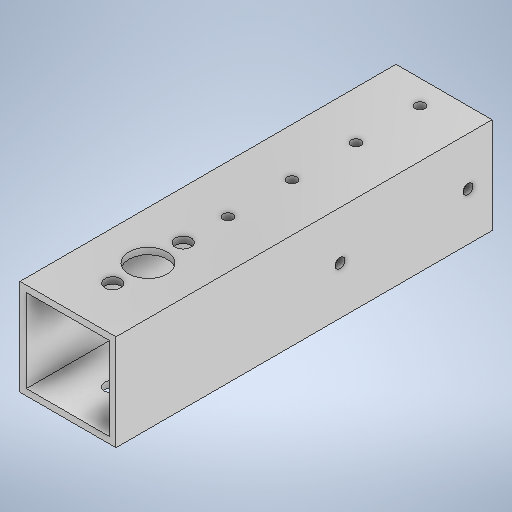
# Autodesk Inventor part: hand2_03
Saved by Autodesk Inventor 2025.1 (Build 291241000, 241)
## iProperties
Created: 2025-02-02
Part Number: hand2_03
Material: アルミニウム 6061-AHC
Document SubType Name: Modeling
Designer: ryogo
Density: 2.7 g/cm^3
Appearance: アルミニウム - ダーク
Author: ryogo
Autodesk Inventor part; units mm, degrees
ref_plane "YZ Plane" through (0, 0, 0) normal (1, 0, 0) x (0, 1, 0)
ref_plane "XZ Plane" through (0, 0, 0) normal (0, 1, 0) x (-1, 0, 0)
ref_plane "XY Plane" through (0, 0, 0) normal (0, 0, 1) x (1, 0, 0)
sketch "スケッチ1" plane through (0, 0, 0) normal (0, 1, 0) x (-1, 0, 0)
  circle A0 centre (0, 0) radius 122.5
  line L0 (0, 0) -> (21.2719, 120.6389)
  line L1 (21.2719, 120.6389) -> (-21.2719, -120.6389)
  line L2 (21.2719, 120.6389) -> (-41.166, -233.4643)
  arc A1 (21.2719, 120.6389) -> (0, 122.5) centre (0, 0) ccw
  arc A2 (-21.2719, -120.6389) -> (0, -122.5) centre (0, 0) ccw
  arc A3 (-41.8975, -115.1123) -> (-21.2719, -120.6389) centre (0, 0) ccw
  circle A4 centre (0, 0) radius 125
  circle A5 centre (0, 0) radius 145
  arc A6 (-42.7525, -117.4616) -> (-105.9051, -66.4011) centre (0, 0) ccw
  line L3 (0, 0) -> (-42.7525, -117.4616) construction
  line L4 (21.706, 123.101) -> (21.706, 123.101)
  line L5 (0, -145) -> (0, -265.735)
  line L6 (0, 0) -> (-41.8975, -115.1123)
  line L7 (-49.5929, -136.2554) -> (-41.8975, -115.1123)
  line L8 (-42.7525, -117.4616) -> (-231.4975, -48.764)
  line L9 (42.7525, 117.4616) -> (0, 0)
  line L10 (0, -145) -> (0, 145)
  line L11 (0, 0) -> (0, 250)
  circle A7 centre (0, 250) radius 20
  line L12 (113.4405, 52.5) -> (18.1505, 258.4)
  line L13 (0, 0) -> (185.4327, 0)
  line L14 (0, 0) -> (-259.4726, 94.4403)
  line L15 (42.7525, 117.4616) -> (-253.7236, 225.3701)
  line L16 (0, 125) -> (22.0409, 125)
  line L17 (21.2719, 120.6389) -> (25.179, 142.7971)
  line L18 (42.7525, 117.4616) -> (60.6365, 166.5974)
  line L19 (15, 170) -> (59.0618, 170)
  line L20 (15.9946, 175) -> (56.7478, 175)
  line L21 (0, 125) -> (-15, 125)
  line L22 (-15, 125) -> (-15, 275)
  line L23 (-15, 275) -> (0, 275)
  line L24 (0, 275) -> (0, 125)
  line L25 (0, 125) -> (15, 125)
  line L26 (15, 125) -> (15, 275)
  line L27 (15, 275) -> (0, 275)
  line L28 (0, 275) -> (0, 125)
  line L29 (15, 200) -> (15, 275)
  line L30 (15, 275) -> (-15, 275)
  line L31 (-15, 275) -> (-15, 150)
  line L32 (15, 170) -> (37.5, 170)
  line L33 (37.5, 170) -> (17.5, 170)
  line L34 (0, 0) -> (0, 250)
  line L35 (0, -125) -> (42.7525, 117.4616)
  line L36 (-42.7525, -117.4616) -> (0, 125)
  line L37 (0, -125) -> (-3.519, -144.9573)
  line L38 (42.7525, 117.4616) -> (49.5929, 136.2554)
  line L39 (0, 125) -> (3.519, 144.9573)
  line L40 (-42.7525, -117.4616) -> (-46.2715, -137.4189)
  line L41 (42.7525, 117.4616) -> (46.2715, 137.4189)
  line L42 (-3.519, -144.9573) -> (46.2715, 137.4189)
  line L43 (46.2715, 137.4189) -> (37.2054, 139.0175)
  line L44 (-12.5852, -143.3587) -> (-3.519, -144.9573)
  line L45 (-46.2715, -137.4189) -> (3.519, 144.9573)
  line L46 (3.519, 144.9573) -> (12.5852, 143.3587)
  line L47 (-37.2054, -139.0175) -> (-46.2715, -137.4189)
  line L48 (-27.6373, -142.3418) -> (-22.7132, -143.21)
  line L49 (-27.6373, -142.3418) -> (-22.7132, -143.21)
  line L50 (-22.7132, -143.21) -> (27.641, 142.363)
  line L51 (27.641, 142.363) -> (22.717, 143.2312)
  line L52 (22.717, 143.2312) -> (-27.6373, -142.3418)
  line L53 (12.5852, 143.3587) -> (-37.2054, -139.0175)
  line L54 (-12.5852, -143.3587) -> (37.2054, 139.0175)
  line L55 (-42.1294, -138.1492) -> (7.6611, 144.2269)
  line L56 (-7.6611, -144.2269) -> (42.1294, 138.1492)
  line L57 (12.5852, 143.3587) -> (7.6611, 144.2269)
  line L58 (7.6611, 144.2269) -> (23.8851, 236.2374)
  line L59 (23.8851, 236.2374) -> (28.8091, 235.3692)
  line L60 (28.8091, 235.3692) -> (12.5852, 143.3587)
  line L61 (22.717, 143.2312) -> (25.179, 142.7971)
  line L62 (25.179, 142.7971) -> (42.462, 240.8141)
  line L63 (42.462, 240.8141) -> (40, 241.2482)
  line L64 (40, 241.2482) -> (22.717, 143.2312)
  line L65 (42.1294, 138.1492) -> (37.2054, 139.0175)
  line L66 (37.2054, 139.0175) -> (45.9435, 188.5741)
  line L67 (45.9435, 188.5741) -> (50.8676, 187.7058)
  line L68 (50.8676, 187.7058) -> (42.1294, 138.1492)
  line L69 (25.179, 142.7971) -> (27.641, 142.363)
  line L70 (27.641, 142.363) -> (39.8383, 211.5375)
  line L71 (39.8383, 211.5375) -> (37.3763, 211.9716)
  line L72 (37.3763, 211.9716) -> (25.179, 142.7971)
  line L73 (15.9946, 175) -> (15, 175)
  line L74 (15, 175) -> (0, 175)
  line L75 (0, 175) -> (0, 170)
  line L76 (0, 170) -> (15, 170)
  line L77 (15, 170) -> (15, 175)
  line L78 (20, 175) -> (40, 175)
  line L79 (40, 175) -> (40, 245)
  line L80 (40, 245) -> (20, 245)
  line L81 (20, 245) -> (20, 175)
  line L82 (30, 175) -> (30, 118.7697)
  line L83 (0, 175) -> (45.1779, 175)
  line L84 (45.1779, 175) -> (45.1779, 200)
  line L85 (45.1779, 200) -> (0, 200)
  line L86 (0, 200) -> (0, 175)
  line L87 (0, 200) -> (50, 200)
  line L88 (50, 200) -> (50, 170)
  line L89 (50, 170) -> (0, 170)
  line L90 (0, 170) -> (0, 200)
  line L91 (50, 170) -> (0, 170)
  line L92 (0, 170) -> (0, 165)
  line L93 (0, 200) -> (-15, 200)
  line L94 (-15, 200) -> (-15, 180)
  line L95 (-15, 180) -> (0, 180)
  line L96 (0, 180) -> (0, 200)
  line L97 (0, 180) -> (-15, 180)
  line L98 (-15, 180) -> (-15, 175)
  line L99 (-15, 175) -> (0, 175)
  line L100 (0, 175) -> (0, 180)
  line L101 (0, 145) -> (-15, 145)
  line L102 (-15, 145) -> (-20.5, 145)
  line L103 (-20.5, 145) -> (-20.5, 200)
  line L104 (-20.5, 200) -> (-15, 200)
  line L105 (-15, 200) -> (-15, 145)
  line L106 (-20.5, 150) -> (-25, 150)
  line L107 (-25, 150) -> (-25, 180)
  line L108 (-25, 180) -> (-20.5, 180)
  line L109 (-20.5, 180) -> (-20.5, 150)
  line L110 (50, 175) -> (-15, 175)
  line L111 (-15, 175) -> (-15, 170)
  line L112 (50, 170) -> (50, 175)
  line L113 (-20.5, 165) -> (-25, 165)
  line L114 (-25, 165) -> (-25, 195)
  line L115 (-25, 195) -> (-20.5, 195)
  line L116 (-20.5, 195) -> (-20.5, 165)
  line L117 (15, 250) -> (-15, 250)
  line L118 (-15, 145) -> (15, 145)
  line L119 (26.3471, 235.8033) -> (-39.6674, -138.5834)
  line L120 (48.4056, 188.14) -> (-10.1232, -143.7928)
  line L121 (49.3441, 179.0659) -> (14.8758, 185.1436)
  line L122 (-15, 138.4818) -> (-15, 121.5782)
  line L123 (-7.6611, -144.2269) -> (-42.1294, -138.1492)
  line L124 (-39.6243, -123.9424) -> (-5.1561, -130.02)
  line L125 (-42.2291, -138.7145) -> (-7.7608, -144.7922)
  line L126 (-41.3608, -133.7904) -> (-6.8926, -139.8681)
  line L127 (-6.0243, -134.9441) -> (-40.4926, -128.8664)
  line L128 (18.3488, 204.8397) -> (52.8171, 198.762)
  line L129 (50.2124, 183.9899) -> (45.0029, 154.4457)
  line L130 (10.5346, 160.5234) -> (15.7441, 190.0676)
  line L131 (19.217, 209.7638) -> (53.6853, 203.6861)
  line L132 (15, 250) -> (53.6853, 203.6861)
  line L133 (53.6853, 203.6861) -> (53.6853, 170)
  line L134 (53.6853, 170) -> (-15, 170)
  line L135 (-15, 172.5) -> (53.6853, 172.5)
  line L136 (15, 170) -> (15, 150)
  line L137 (15, 150) -> (-15, 150)
  line L138 (-15, 170) -> (15, 170)
  line L139 (15, 150) -> (-15, 150)
  line L140 (-15, 150) -> (-15, 275)
  line L141 (-15, 275) -> (15, 275)
  line L142 (15, 275) -> (15, 150)
  circle A8 centre (0, 250) radius 6
  circle A9 centre (0, 250) radius 11
  line L143 (47.7456, 170) -> (15, 150)
  point P0 (-25.1752, -142.7759)
  point P1 (42.3116, 114.9608)
  point P2 (0, 133.0222)
  point P3 (-38.8988, -134.2246)
  point P4 (-38.0306, -129.3005)
  point P5 (-23.2585, -131.9052)
  point P6 (-24.1267, -136.8293)
  point P7 (-9.3546, -139.434)
  point P8 (-8.4863, -134.51)
  point P9 (17.3379, 184.7094)
  point P10 (32.11, 182.1047)
  point P11 (46.8821, 179.5)
  point P12 (50.3551, 199.1962)
  point P13 (35.5829, 201.8009)
  point P14 (20.8108, 204.4056)
  point P15 (0, 240)
  point P16 (0, 190)
  point P17 (0, 239)
  point P18 (0, 261)
  point P19 (37.5, 172.5)
  point P20 (22.5, 172.5)
  point P21 (0, 275)
  point P22 (15, 185.1217)
  point P23 (15, 185.8477)
  point P24 (-11, 250)
  point P25 (11, 250)
  dimension "d0" = 245
  dimension "d7" = 290
  dimension "d19" = 40
  dimension "d1" = 0
  dimension "d4" = 42.5438
  dimension "d5" = 21.3532
  dimension "d6" = 250
  dimension "d10" = 0
  dimension "d12" = 0
  dimension "d13" = 10
  dimension "d15" = 0
  dimension "d16" = 9.8877
  dimension "d18" = 10
  dimension "d21" = 145
  dimension "d23" = 125
  dimension "d26" = 7.5384
  dimension "d30" = 180
  dimension "d34" = 180
  dimension "d35" = 45
  dimension "d37" = 5
  dimension "d38" = 15
  dimension "d39" = 150
  dimension "d40" = 15
  dimension "d41" = 150
  dimension "d47" = 250
  dimension "d52" = 5
  dimension "d53" = 0
  dimension "d54" = 10
  dimension "d55" = 10
  dimension "d56" = 5
  dimension "d57" = 5
  dimension "d60" = 5
  dimension "d61" = 20
  dimension "d62" = 70
  dimension "d63" = 5
  dimension "d65" = 25
  dimension "d66" = 50
  dimension "d68" = 20
  dimension "d69" = 5
  dimension "d74" = 20
  dimension "d75" = 5.5
  dimension "d76" = 55
  dimension "d77" = 4.5
  dimension "d78" = 30
  dimension "d79" = 5
  dimension "d82" = 15
  dimension "d83" = 50
  dimension "d87" = 16.9036
  dimension "d88" = 10.0392
  dimension "d89" = 10.5222
  dimension "d92" = 15
  dimension "d93" = 5
  dimension "d94" = 5
  dimension "d96" = 4.5
  dimension "d97" = 5
  dimension "d98" = 30
  dimension "d99" = 10
  dimension "d101" = 20
  dimension "d102" = 10
  dimension "d103" = 20
  dimension "d104" = 12
  dimension "d105" = 22
  dimension "d106" = 7.5
  dimension "d107" = 15
  dimension "d108" = 30
  constraints: 287 end point, 86 point on line, 44 parallel, 39 perpendicular, 19 horizontal, 18 point on circle, 15 midpoint, 9 coincident, 9 collinear, 7 centre point, 3 vertical, 2 tangent, 1 symmetric about line, 43 other
  measures "d1" horizontal distance of point (0, 0) A2.end
  measures "d4" distance of L6.end A2.end
  measures "d5" distance of A1.end L0.end
  measures "d6" diameter of A4
  measures "d10" horizontal distance of A4.centre L16.start
  measures "d12" distance from line of L5 point (0, 0)
  measures "d15" horizontal distance of A2.end L35.start
  measures "d16" vertical distance of L6.end L35.start
  measures "d18" angle of L9 L1
  measures "d21" distance of L5.start A2.centre
  measures "d23" distance of L11.end L16.start
  measures "d26" distance from line of L15 L16.start
  measures "d30" angle of L4 L17
  measures "d34" angle of L9 L18
  measures "d35" distance from line of L19 L16.start
  measures "d37" distance between parallel lines of L19 L20
  measures "d38" distance of L22.end L23.end
  measures "d39" distance of L21.end L22.end
  measures "d40" distance of L27.end L26.end
  measures "d41" distance from line of L16.start L27
  measures "d47" distance of L3.start L11.end
  measures "d52" distance of L48.start L48.end
  measures "d53" distance from line of L2 point (-25.175, -142.776)
  measures "d54" distance between parallel lines of L52 L53
  measures "d55" distance between parallel lines of L54 L50
  measures "d56" distance of L46.end L55.end
  measures "d57" distance of L43.end L56.end
  measures "d60" distance between parallel lines of L76 L74
  measures "d61" distance of L80.end L79.end
  measures "d62" distance of L79.end L78.end
  measures "d63" distance between parallel lines of L26 L81
  measures "d65" distance of L84.end L83.end
  measures "d66" distance of L88.end L89.end
  measures "d68" distance between parallel lines of L95 L93
  measures "d69" distance between parallel lines of L99 L97
  measures "d74" distance of L16.start L101.start
  measures "d75" distance of L103.end L104.end
  measures "d76" distance of L102.end L103.end
  measures "d77" distance of L107.end L108.end
  measures "d78" distance of L106.end L107.end
  measures "d79" distance between parallel lines of L102 L106
  measures "d82" distance between parallel lines of L106 L113
  measures "d83" distance between parallel lines of L93 L117
  measures "d87" distance of L122.start L122.end
  measures "d88" vertical distance of point (42.312, 114.961) L25.end
  measures "d89" distance of A1.end point (0, 133.022)
  measures "d92" distance of L125.start L124.start
  measures "d93" distance of L125.start L126.start
  measures "d94" distance of L127.end L124.start
  measures "d96" distance from line of L20 point (46.882, 179.5)
  measures "d97" distance of L121.end L130.end
  measures "d98" distance of L129.start L129.end
  measures "d99" distance from line of L117 point (0, 240)
  measures "d101" distance of L128.start L121.end
  measures "d102" diameter of L131 L128
  measures "d103" distance of L19.start L136.end
  measures "d104" diameter of A8
  measures "d105" diameter of A9
  measures "d106" distance from line of point (22.5, 172.5) L142
  measures "d107" distance of point (22.5, 172.5) point (37.5, 172.5)
  measures "d108" distance between parallel lines of L113 L115
extrude "押し出し1" add sketch "スケッチ1" along normal blind 30 contours L137 L60 L26 | L60 L137 L119 L76 L26 | L76 L119 L26 | L137 L58 L76 L119 | L119 L76 L58 L135 L26 | L137 L11 L76 L58 | L26 L117 A9 L24 A7 | A7 L24 L27 L26 | L137 L22 L134 L11 | L135 L58 L74 L26 | L76 L11 L135 L58 | L24 A9 L117 L22 A7 | A7 L22 L23 L24 | L26 A7 L11 A9 L117 | L74 L58 L121 L26 | L135 L11 L74 L58 | L134 L22 L135 L11 | L26 L85 L11 A7 | A9 L117 A8 L24 | L24 A8 L117 A9 | A9 L11 A8 L117 | L121 L58 L26 | L74 L11 L85 L26 L58 | L135 L22 L99 L11 | A7 L22 L117 A9 L11 | L11 L93 L22 A7 | L117 A8 L11 A9 | L99 L22 L95 L11 | L11 L95 L22 L93
shell "シェル1" thickness 2 removed faces 3 at (-5, 10, 275) at (-5.9805, 20, 249.5172) at (5, 10, 150)
sketch "スケッチ3" plane through (0, 0, 0) normal (0, -1, 0) x (1, 0, 0)
  line L0 (15, 150) -> (-15, 150) projected
  line L1 (-13, 150) -> (-13, 275) projected
  point P0 (0, 0)
  point P1 (0, 165)
  point P2 (0, 150)
  point P3 (0, 240)
  point P4 (0, 185)
  point P5 (0, 205)
  point P6 (0, 225)
  dimension "d119" = 15
  dimension "d120" = 0
  dimension "d146" = 20
  dimension "d147" = 20
  dimension "d148" = 13
  dimension "d151" = 20
  constraints: 1 midpoint
  measures "d119" distance from line of L0 point (0, 165)
  measures "d120" horizontal distance of point (0, 150) point (0, 165)
  measures "d146" distance of point (0, 165) point (0, 185)
  measures "d147" distance of point (0, 205) point (0, 185)
  measures "d148" distance from line of L1 point (0, 205)
  measures "d151" distance of point (0, 225) point (0, 205)
hole "穴1" at (0, 0, 239) at (0, 0, 261) direction (0, 1, 0) diameter 5 end through all
hole "穴2" at (0, 0, 165) at (0, 0, 240) at (0, 0, 205) at (0, 0, 185) at (0, 0, 225) direction (0, 1, 0) diameter 3.1 end through all
sketch "スケッチ4" plane through (-15, 0, 150) normal (-1, 0, 0) x (0, 0, 1)
  line L0 (0, 0) -> (0, 30) projected
  line L1 (0, 15) -> (125, 15)
  line L2 (125, 0) -> (125, 30) projected
  point P0 (-150, 0)
  point P1 (15, 15)
  point P2 (55, 15)
  dimension "d129" = 15
  dimension "d130" = 40
  constraints: 2 end point, 2 midpoint, 2 point on line
  measures "d129" distance from line of L0 point (15, 15)
  measures "d130" distance of point (55, 15) point (15, 15)
hole "穴3" at (-15, 15, 165) at (-15, 15, 205) direction (1, 0, 0) diameter 3.1 end through all
sketch "スケッチ6" plane through (-15, 0, 150) normal (-1, 0, 0) x (0, 0, 1)
  circle A0 centre (15, 15) radius 1.55 projected
  circle A1 centre (15, 15) radius 5
  circle A2 centre (55, 15) radius 1.55 projected
  circle A3 centre (55, 15) radius 5
  point P0 (-150, 0)
  dimension "d142" = 10
  dimension "d143" = 10
  constraints: 2 centre point, 2 coincident
  measures "d142" diameter of A1
  measures "d143" diameter of A3
extrude "押し出し3" cut sketch "スケッチ6" against normal blind 5 contours A0 | A1 | A2 | A3
sketch "スケッチ7" plane through (15, 0, 150) normal (0, 0, -1) x (-1, 0, 0)
  line L0 (2, 2) -> (2, 28) projected
  line L1 (2, 28) -> (28, 28) projected
  line L2 (28, 28) -> (28, 2) projected
  line L3 (28, 2) -> (2, 2) projected
  line L4 (0, 0) -> (30, 0) projected
  line L5 (30, 0) -> (30, 30) projected
  line L6 (0, 30) -> (30, 30) projected
  line L7 (0, 0) -> (0, 30) projected
  point P0 (15, 0)
extrude "押し出し4" cut sketch "スケッチ7" against normal blind 7.5
equation "\"d18\" = d13"
